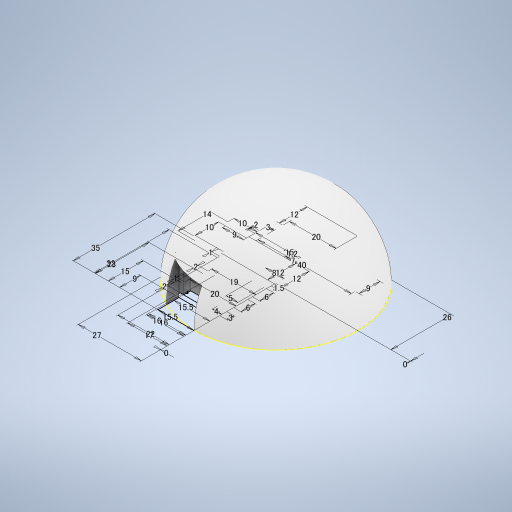
# Autodesk Inventor part: naibu
Saved by Autodesk Inventor 2023 (Build 270158000, 158)
## iProperties
Created: 2022-10-08
Part Number: naibu
Material: ABS プラスチック
Document SubType Name: Modeling
Designer: ellie
Density: 1.06 g/cm^3
Appearance: 積雪
Author: ellie
Autodesk Inventor part; units mm, degrees
ref_plane "YZ Plane" through (0, 0, 0) normal (1, 0, 0) x (0, 1, 0)
ref_plane "XZ Plane" through (0, 0, 0) normal (0, 1, 0) x (-1, 0, 0)
ref_plane "XY Plane" through (0, 0, 0) normal (0, 0, 1) x (1, 0, 0)
sketch "スケッチ1" plane through (0, 0, 0) normal (0, 1, 0) x (-1, 0, 0)
  circle A0 centre (0, 0) radius 35
  line L0 (0, 0) -> (0, -35)
  line L1 (0, 0) -> (0, 35)
  dimension "d0" = 70
  constraints: 4 end point, 2 point on circle, 2 vertical, 1 centre point, 1 coincident
  measures "d0" diameter of A0
revolve "回転1" add sketch "スケッチ1" angle 180 about axis through (0, 0, 0) along (0, 0, 1) picked at (-2.5961, -23.0408) contours L1 L0 A0
sketch "スケッチ5" plane through (0, 0, 0) normal (0, -1, 0) x (1, 0, 0)
  line L0 (-20, -23) -> (20, -23)
  line L1 (20, -23) -> (20, -14)
  line L2 (20, -14) -> (-20, -14)
  line L3 (-20, -14) -> (-20, -23)
  line L4 (-20, -14) -> (-23, -14)
  line L5 (-23, -14) -> (-23, -16)
  line L6 (-23, -16) -> (-20, -16)
  line L7 (-20, -16) -> (-20, -14)
  line L8 (0, 26) -> (-17, 26)
  line L9 (-17, 26) -> (-17, 24)
  line L10 (-17, 24) -> (0, 24)
  line L11 (0, 24) -> (0, 26)
  line L12 (0, 20) -> (-20, 20)
  line L13 (-20, 20) -> (-20, 19)
  line L14 (-20, 19) -> (0, 19)
  line L15 (0, 19) -> (0, 20)
  line L16 (0, 12) -> (-19, 12)
  line L17 (-19, 12) -> (-19, 10)
  line L18 (-19, 10) -> (0, 10)
  line L19 (0, 10) -> (0, 12)
  line L20 (0, 3) -> (-22, 3)
  line L21 (-22, 3) -> (-22, 2)
  line L22 (-22, 2) -> (0, 2)
  line L23 (0, 2) -> (0, 3)
  circle A0 centre (0, 0) radius 35 projected
  circle A1 centre (0, 0) radius 35 projected
  line L24 (0, 35) -> (0, -35)
  line L25 (35, 0) -> (-35, 0)
  line L26 (-32, -0.5) -> (-23, -0.5)
  line L27 (-23, -0.5) -> (-23, -10.5)
  line L28 (-23, -10.5) -> (-32, -10.5)
  line L29 (-32, -10.5) -> (-32, -0.5)
  line L30 (-23, -8.0262) -> (-23, -0.5)
  line L31 (-27, 22.2711) -> (-27, -22.2711)
  line L32 (-15.5, 26) -> (0, 26)
  line L33 (0, 26) -> (0, 35)
  line L34 (0, 35) -> (-15.5, 35)
  line L35 (-15.5, 35) -> (-15.5, 26)
  line L36 (-15.5, 24) -> (0, 24)
  line L37 (0, 24) -> (0, 21)
  line L38 (0, 21) -> (-15.5, 21)
  line L39 (-15.5, 21) -> (-15.5, 24)
  line L40 (-16, 12) -> (0, 12)
  line L41 (0, 12) -> (0, 18)
  line L42 (0, 18) -> (-16, 18)
  line L43 (-16, 18) -> (-16, 12)
  line L44 (-16, 10) -> (0, 10)
  line L45 (0, 10) -> (0, 4)
  line L46 (0, 4) -> (-16, 4)
  line L47 (-16, 4) -> (-16, 10)
  line L48 (-23, -5.5) -> (-39.6865, -5.5)
  line L49 (-23, -5.5) -> (-7.8337, -5.5)
  line L50 (-8, 0.5) -> (-23, 0.5)
  line L51 (-23, 0.5) -> (-23, -11.5)
  line L52 (-23, -11.5) -> (-8, -11.5)
  line L53 (-8, -11.5) -> (-8, 0.5)
  line L54 (-8, 0.5) -> (-23, -11.5) construction
  line L55 (-23, 0.5) -> (-8, -11.5) construction
  line L56 (-23, 1.5) -> (-33, 1.5)
  line L57 (-33, 1.5) -> (-33, -12.5)
  line L58 (-33, -12.5) -> (-23, -12.5)
  line L59 (-23, -12.5) -> (-23, 1.5)
  line L60 (-23, 1.5) -> (-33, -12.5) construction
  line L61 (-33, 1.5) -> (-23, -12.5) construction
  line L62 (-8, 0.5) -> (-1, 0.5)
  line L63 (-1, 0.5) -> (-1, -11.5)
  line L64 (-1, -11.5) -> (-8, -11.5)
  line L65 (-8, -11.5) -> (-8, 0.5)
  line L66 (-8, 0.5) -> (-1, -11.5) construction
  line L67 (-1, 0.5) -> (-8, -11.5) construction
  line L68 (-23, -0.5) -> (-27, -0.5)
  line L69 (-23, -10.5) -> (-27, -10.5)
  line L70 (-23, 1.5) -> (-27, 1.5)
  line L71 (-23, -12.5) -> (-27, -12.5)
  line L72 (23.4307, -26) -> (-23.4307, -26)
  line L73 (-8, 0.5) -> (-6.8, 0.5)
  line L74 (-6.8, 0.5) -> (-6.8, -11.5)
  line L75 (-6.8, -11.5) -> (-8, -11.5)
  line L76 (-8, -11.5) -> (-8, 0.5)
  line L77 (-2, 4) -> (1, 4)
  line L78 (-1, -8) -> (-1, -4)
  line L79 (0, 21) -> (-4, 21)
  line L80 (-4, 21) -> (-4, 18)
  line L81 (-4, 18) -> (0, 18)
  line L82 (0, 18) -> (0, 21)
  line L83 (-6, 4) -> (-1, 4)
  line L84 (-1, 4) -> (-1, 0.5)
  line L85 (-1, 0.5) -> (-6, 0.5)
  line L86 (-6, 0.5) -> (-6, 4)
  point P0 (0, -23)
  point P1 (0, -14)
  point P2 (-20, -16)
  point P3 (0, 25)
  point P4 (0, 19.5)
  point P5 (0, 11)
  point P6 (0, 2.5)
  point P7 (-20, -18.5)
  point P8 (-27, -0.5262)
  point P9 (-27, -10.5)
  point P10 (-15.5, 22.5)
  point P11 (-15.5, 31.3807)
  point P12 (0, 26)
  point P13 (0, 24)
  point P14 (0, 10)
  point P15 (0, 12)
  point P16 (-27, 0)
  point P17 (-29, 0)
  point P18 (-20, 0)
  point P19 (-15.5, -5.5)
  point P20 (-28, -5.5)
  point P21 (-4.5, -5.5)
  point P22 (-8, -11.5)
  point P23 (-8, 0.5)
  point P24 (-27, 0.5)
  point P25 (-28, 0.4738)
  point P26 (-28, -11.5262)
  point P27 (-27, -11.5)
  point P28 (-23, -10.5)
  point P29 (-23, -0.5)
  point P30 (-23, -0.5)
  point P31 (-23, -10.5)
  point P32 (-23, 0.5)
  point P33 (-23, -11.5)
  point P34 (-8, 0)
  point P35 (-1, 0)
  point P36 (-8, -11.5)
  point P37 (-4, 19)
  point P38 (0, 19)
  point P39 (-4, 20)
  point P40 (0, 20)
  point P41 (-1, 0.5)
  point P42 (-1, 4)
  dimension "d12" = 40
  dimension "d13" = 9
  dimension "d21" = 3
  dimension "d22" = 2
  dimension "d23" = 17
  dimension "d24" = 2
  dimension "d27" = 20
  dimension "d28" = 1
  dimension "d30" = 19
  dimension "d31" = 2
  dimension "d33" = 1
  dimension "d88" = 0
  dimension "d89" = 0
  dimension "d90" = 12
  dimension "d92" = 20
  dimension "d93" = 9
  dimension "d94" = 15
  dimension "d95" = 23
  dimension "d96" = 32
  dimension "d97" = 9
  dimension "d98" = 10
  dimension "d113" = 27
  dimension "d122" = 15.5
  dimension "d123" = 35
  dimension "d124" = 3
  dimension "d125" = 15.5
  dimension "d126" = 6
  dimension "d127" = 6
  dimension "d128" = 16
  dimension "d129" = 16
  dimension "d137" = 22
  dimension "d147" = 12
  dimension "d148" = 1.5
  dimension "d149" = 8
  dimension "d151" = 15
  dimension "d161" = 14
  dimension "d162" = 10
  dimension "d164" = 12
  dimension "d165" = 7
  dimension "d170" = 26
  dimension "d175" = 1.2
  dimension "d195" = 4
  dimension "d201" = 5
  constraints: 172 end point, 35 parallel, 21 horizontal, 20 perpendicular, 17 point on line, 15 midpoint, 6 collinear, 1 vertical, 20 other
  measures "d12" distance of L2.end L1.end
  measures "d13" distance of L1.end L0.end
  measures "d21" distance of L6.end L5.end
  measures "d22" distance of L5.end L4.end
  measures "d23" distance of L10.end L9.end
  measures "d24" distance of L9.end L8.end
  measures "d27" distance of L14.end L13.end
  measures "d28" distance of L13.end L12.end
  measures "d30" distance of L18.end L17.end
  measures "d31" distance of L17.end L16.end
  measures "d33" distance of L21.end L20.end
  measures "d89" distance from line of point (0, 0) L25
  measures "d90" distance from line of L0 point (0, -35)
  measures "d92" distance of the line from the sketch origin of L3
  measures "d93" distance from line of L8 point (0, 35)
  measures "d94" distance from line of L12 point (0, 35)
  measures "d95" distance from line of L16 point (0, 35)
  measures "d96" distance from line of L20 point (0, 35)
  measures "d97" distance of L27.end L28.end
  measures "d98" distance of L26.end L27.end
  measures "d113" distance of the line from the sketch origin of L31
  measures "d122" distance of the line from the sketch origin of L35
  measures "d123" distance between parallel lines of L34 L25
  measures "d124" distance of L36.end L37.end
  measures "d126" distance of L41.end L40.end
  measures "d127" distance of L44.end L45.end
  measures "d128" distance of the line from the sketch origin of L47
  measures "d129" distance of the line from the sketch origin of L43
  measures "d137" distance of L21.end L22.end
  measures "d147" distance of L51.end L50.end
  measures "d148" distance between parallel lines of L50 L22
  measures "d149" distance of the line from the sketch origin of L53
  measures "d151" distance between parallel lines of L53 L27
  measures "d161" distance between parallel lines of L58 L56
  measures "d162" distance between parallel lines of L51 L57
  measures "d164" distance between parallel lines of L64 L62
  measures "d165" distance between parallel lines of L53 L63
  measures "d170" distance between parallel lines of L72 L25
  measures "d175" distance of L74.end L75.end
  measures "d195" distance of the line from the sketch origin of L80
  measures "d201" distance between parallel lines of L84 L86
extrude "GNSボード" cut sketch "スケッチ5" against normal blind 16 contours L11 L10 L9 L8
extrude "GNSボード止めるよう" cut sketch "スケッチ5" against normal blind 15 contours L24 L8 L35 A0 | L24 L38 L39 L10
extrude "アルミ板１" cut sketch "スケッチ5" against normal blind 20 contours L15 L14 L80 L12 | L80 L14 L13 L12
extrude "メイン基板" cut sketch "スケッチ5" against normal blind 17.5 contours L18 L17 L16 L19
extrude "メイン止めるよう" cut sketch "スケッチ5" against normal blind 16.5 contours L46 L47 L18 L24 | L16 L43 L42 L24
extrude "アルミ板２" cut sketch "スケッチ5" against normal blind 17.5 contours L22 L84 L20 L23 | L22 L86 L20 L84 | L22 L21 L20 L86
extrude "電池ボックス入れ" cut sketch "スケッチ5" against normal blind 15 contours L3 L2 L24 L0 | L24 L2 L1 L0 | L6 L5 L4 L3
extrude "side ut" cut sketch "スケッチ5" against normal blind 100 contours A0 L58 L31 | A0 L57 L48 L29 L28 L31 L58 | A0 L48 L57 | L28 L29 L48 L31 | L31 L56 L57 L25 A0 | A0 L25 L57 L48 | L57 L25 L31 L26 L29 L48 | L48 L29 L26 L31 | L31 L25 L57 L56
extrude "motor case" add sketch "スケッチ5" against normal blind 7 contours L58 L57 A0 | A0 L57 L48 L29 L28 L31 L58 | L31 L28 L51 L59 L58 | L53 L49 L27 L51 L25 | L25 L51 L50 L53 | L31 L48 L27 L28 | L28 L29 L48 L31 | L51 L26 L31 L25 | L25 L31 L56 L59 L51 | L53 L52 L51 L27 L49 | L57 L25 L31 L26 L29 L48 | L48 L29 L26 L31 | L31 L26 L27 L48 | L31 L25 L57 L56
extrude "bottom cut" cut sketch "スケッチ5" against normal blind 90 contours L72 A0 L24 | L24 A0 L72
extrude "motor" cut sketch "スケッチ5" against normal blind 6 contours L63 L64 L74 L25 | L25 L74 L62 L63 | L74 L64 L53 L25 | L25 L53 L62 L74 | L53 L49 L27 L51 L25 | L25 L51 L50 L53 | L31 L48 L27 L28 | L28 L29 L48 L31 | L53 L52 L51 L27 L49 | L48 L29 L26 L31 | L31 L26 L27 L48
extrude "motor block" add sketch "スケッチ5" against normal blind 10 contours L74 L64 L53 L25 | L25 L53 L62 L74
extrude "押し出し35" cut sketch "スケッチ5" against normal blind 5 contours L24 L12 L80 L38 | L42 L80 L14 L24
mirror "ミラー12" about plane through (0, 0, 0) normal (1, 0, 0) of "押し出し35"
sketch "スケッチ27" plane through (-33, 0, -12.5) normal (-1, 0, 0) x (0, 0, 1)
  line L0 (14, 0) -> (0, 0) projected
  circle A0 centre (7, 0) radius 3
  point P0 (12.5, 0)
  dimension "d198" = 6
  constraints: 1 centre point, 1 midpoint
  measures "d198" diameter of A0
extrude "押し出し36" cut sketch "スケッチ27" against normal blind 27
extrude "押し出し37" cut sketch "スケッチ5" against normal blind 15 contours L84 L62 L86 L22 | L22 L86 L20 L84 | L20 L86 L46 L84
